Autodesk Fusion 360 part; units mm, degrees
note: some values were not read from the file. Set by a fixed rule: the direction of a hole.
(part 3 of 10)
  line L1913 (9.2464, 17.0934) -> (9.2464, 17.0934)
  line L1914 (9.1415, 16.1798) -> (9.1415, 16.1798)
  line L1915 (9.1415, 16.8402) -> (9.1415, 16.8402)
  line L1916 (10.7434, 17.4236) -> (10.6273, 17.5013)
  line L1917 (11.1785, 16.1798) -> (11.1785, 16.1798)
  line L1918 (9.1415, 16.8402) -> (9.1415, 16.1798)
  line L1919 (9.1415, 16.1798) -> (9.1687, 16.0427)
  line L1920 (9.1687, 16.0427) -> (9.2464, 15.9266)
  line L1921 (9.2464, 15.9266) -> (9.2464, 15.9266)
  line L1922 (46.9384, 15.5964) -> (46.9384, 15.5964)
  line L1923 (46.0248, 17.5285) -> (45.8877, 17.5013)
  line L1924 (45.8877, 17.5013) -> (45.7716, 17.4236)
  line L1925 (47.3463, 16.0427) -> (47.3735, 16.1798)
  line L1926 (46.6852, 17.5285) -> (46.6852, 17.5285)
  line L1927 (46.9384, 17.4236) -> (46.8223, 17.5013)
  line L1928 (47.2686, 17.0934) -> (47.2686, 17.0934)
  line L1929 (47.2686, 15.9266) -> (47.3463, 16.0427)
  line L1930 (45.3365, 16.8402) -> (45.3365, 16.8402)
  line L1931 (46.0248, 15.4915) -> (46.6852, 15.4915)
  line L1932 (47.3735, 16.1798) -> (47.3735, 16.8402)
  line L1933 (45.7716, 17.4236) -> (45.4414, 17.0934)
  line L1934 (45.7716, 15.5964) -> (45.8877, 15.5187)
  line L1935 (45.7716, 17.4236) -> (45.7716, 17.4236)
  line L1936 (46.0248, 15.4915) -> (46.0248, 15.4915)
  line L1937 (45.3365, 16.1798) -> (45.3365, 16.1798)
  line L1938 (46.6852, 15.4915) -> (46.6852, 15.4915)
  line L1939 (46.6852, 17.5285) -> (46.0248, 17.5285)
  line L1940 (46.8223, 17.5013) -> (46.6852, 17.5285)
  line L1941 (45.3637, 16.9773) -> (45.3365, 16.8402)
  line L1942 (46.9384, 15.5964) -> (47.2686, 15.9266)
  line L1943 (47.3463, 16.9773) -> (47.2686, 17.0934)
  line L1944 (47.2686, 17.0934) -> (46.9384, 17.4236)
  line L1945 (46.0248, 17.5285) -> (46.0248, 17.5285)
  line L1946 (45.3365, 16.1798) -> (45.3637, 16.0427)
  line L1947 (45.4414, 17.0934) -> (45.4414, 17.0934)
  line L1948 (45.4414, 17.0934) -> (45.3637, 16.9773)
  line L1949 (47.3735, 16.8402) -> (47.3463, 16.9773)
  line L1950 (45.3637, 16.0427) -> (45.4414, 15.9266)
  line L1951 (46.6852, 15.4915) -> (46.8223, 15.5187)
  line L1952 (45.3365, 16.8402) -> (45.3365, 16.1798)
  line L1953 (47.3735, 16.1798) -> (47.3735, 16.1798)
  line L1954 (45.8877, 15.5187) -> (46.0248, 15.4915)
  line L1955 (46.8223, 15.5187) -> (46.9384, 15.5964)
  line L1956 (47.3735, 16.8402) -> (47.3735, 16.8402)
  line L1957 (46.9384, 17.4236) -> (46.9384, 17.4236)
  line L1958 (47.2686, 15.9266) -> (47.2686, 15.9266)
  line L1959 (45.4414, 15.9266) -> (45.4414, 15.9266)
  line L1960 (45.4414, 15.9266) -> (45.7716, 15.5964)
  line L1961 (45.7716, 15.5964) -> (45.7716, 15.5964)
  line L1962 (11.0736, 29.8966) -> (11.0736, 29.8966)
  line L1963 (10.7434, 29.5664) -> (11.0736, 29.8966)
  line L1964 (11.0736, 31.0634) -> (11.0736, 31.0634)
  line L1965 (10.7434, 29.5664) -> (10.7434, 29.5664)
  line L1966 (11.1785, 30.8102) -> (11.1785, 30.8102)
  line L1967 (9.1415, 30.1498) -> (9.1415, 30.1498)
  line L1968 (10.7434, 31.3936) -> (10.7434, 31.3936)
  line L1969 (9.5766, 31.3936) -> (9.5766, 31.3936)
  line L1970 (9.5766, 31.3936) -> (9.2464, 31.0634)
  line L1971 (10.6273, 31.4713) -> (10.4902, 31.4985)
  line L1972 (10.4902, 31.4985) -> (10.4902, 31.4985)
  line L1973 (9.2464, 31.0634) -> (9.2464, 31.0634)
  line L1974 (9.8298, 31.4985) -> (9.6927, 31.4713)
  line L1975 (9.1415, 30.1498) -> (9.1687, 30.0127)
  line L1976 (9.2464, 29.8966) -> (9.2464, 29.8966)
  line L1977 (11.1513, 30.0127) -> (11.1785, 30.1498)
  line L1978 (9.1687, 30.0127) -> (9.2464, 29.8966)
  line L1979 (9.1415, 30.8102) -> (9.1415, 30.1498)
  line L1980 (11.0736, 29.8966) -> (11.1513, 30.0127)
  line L1981 (11.1785, 30.1498) -> (11.1785, 30.1498)
  line L1982 (10.4902, 31.4985) -> (9.8298, 31.4985)
  line L1983 (9.2464, 31.0634) -> (9.1687, 30.9473)
  line L1984 (10.7434, 31.3936) -> (10.6273, 31.4713)
  line L1985 (9.8298, 31.4985) -> (9.8298, 31.4985)
  line L1986 (9.6927, 31.4713) -> (9.5766, 31.3936)
  line L1987 (9.1415, 30.8102) -> (9.1415, 30.8102)
  line L1988 (9.1687, 30.9473) -> (9.1415, 30.8102)
  line L1989 (11.0736, 31.0634) -> (10.7434, 31.3936)
  line L1990 (9.5766, 29.5664) -> (9.5766, 29.5664)
  line L1991 (9.2464, 29.8966) -> (9.5766, 29.5664)
  line L1992 (10.6273, 29.4887) -> (10.7434, 29.5664)
  line L1993 (9.5766, 29.5664) -> (9.6927, 29.4887)
  line L1994 (10.4902, 29.4615) -> (10.4902, 29.4615)
  line L1995 (9.8298, 29.4615) -> (10.4902, 29.4615)
  line L1996 (9.8298, 29.4615) -> (9.8298, 29.4615)
  line L1997 (9.6927, 29.4887) -> (9.8298, 29.4615)
  line L1998 (10.4902, 29.4615) -> (10.6273, 29.4887)
  line L1999 (11.1513, 30.9473) -> (11.0736, 31.0634)
  line L2000 (11.1785, 30.8102) -> (11.1513, 30.9473)
  line L2001 (11.1785, 30.1498) -> (11.1785, 30.8102)
  line L2002 (56.1315, 16.8402) -> (56.1315, 16.8402)
  line L2003 (56.5666, 17.4236) -> (56.5666, 17.4236)
  line L2004 (56.5666, 17.4236) -> (56.2364, 17.0934)
  line L2005 (56.8198, 17.5285) -> (56.6827, 17.5013)
  line L2006 (57.6173, 15.5187) -> (57.7334, 15.5964)
  line L2007 (58.1685, 16.1798) -> (58.1685, 16.1798)
  line L2008 (58.0636, 17.0934) -> (57.7334, 17.4236)
  line L2009 (57.7334, 17.4236) -> (57.7334, 17.4236)
  line L2010 (56.8198, 17.5285) -> (56.8198, 17.5285)
  line L2011 (57.6173, 17.5013) -> (57.4802, 17.5285)
  line L2012 (58.0636, 15.9266) -> (58.0636, 15.9266)
  line L2013 (56.2364, 17.0934) -> (56.1587, 16.9773)
  line L2014 (56.1315, 16.1798) -> (56.1587, 16.0427)
  line L2015 (56.1315, 16.1798) -> (56.1315, 16.1798)
  line L2016 (57.7334, 17.4236) -> (57.6173, 17.5013)
  line L2017 (57.7334, 15.5964) -> (58.0636, 15.9266)
  line L2018 (58.1685, 16.8402) -> (58.1685, 16.8402)
  line L2019 (58.1685, 16.1798) -> (58.1685, 16.8402)
  line L2020 (56.8198, 15.4915) -> (57.4802, 15.4915)
  line L2021 (58.1685, 16.8402) -> (58.1413, 16.9773)
  line L2022 (58.1413, 16.9773) -> (58.0636, 17.0934)
  line L2023 (58.0636, 15.9266) -> (58.1413, 16.0427)
  line L2024 (58.0636, 17.0934) -> (58.0636, 17.0934)
  line L2025 (58.1413, 16.0427) -> (58.1685, 16.1798)
  line L2026 (57.4802, 15.4915) -> (57.6173, 15.5187)
  line L2027 (57.4802, 15.4915) -> (57.4802, 15.4915)
  line L2028 (56.1315, 16.8402) -> (56.1315, 16.1798)
  line L2029 (56.1587, 16.9773) -> (56.1315, 16.8402)
  line L2030 (56.1587, 16.0427) -> (56.2364, 15.9266)
  line L2031 (56.2364, 17.0934) -> (56.2364, 17.0934)
  line L2032 (57.4802, 17.5285) -> (56.8198, 17.5285)
  line L2033 (56.6827, 15.5187) -> (56.8198, 15.4915)
  line L2034 (56.6827, 17.5013) -> (56.5666, 17.4236)
  line L2035 (56.5666, 15.5964) -> (56.6827, 15.5187)
  line L2036 (56.5666, 15.5964) -> (56.5666, 15.5964)
  line L2037 (57.7334, 15.5964) -> (57.7334, 15.5964)
  line L2038 (56.8198, 15.4915) -> (56.8198, 15.4915)
  line L2039 (56.2364, 15.9266) -> (56.5666, 15.5964)
  line L2040 (57.4802, 17.5285) -> (57.4802, 17.5285)
  line L2041 (56.2364, 15.9266) -> (56.2364, 15.9266)
  line L2042 (21.8687, 19.8527) -> (21.9464, 19.7366)
  line L2043 (21.9464, 20.9034) -> (21.9464, 20.9034)
  line L2044 (22.2766, 21.2336) -> (21.9464, 20.9034)
  line L2045 (21.9464, 20.9034) -> (21.8687, 20.7873)
  line L2046 (22.3927, 21.3113) -> (22.2766, 21.2336)
  line L2047 (22.2766, 21.2336) -> (22.2766, 21.2336)
  line L2048 (23.4434, 21.2336) -> (23.3273, 21.3113)
  line L2049 (22.5298, 21.3385) -> (22.3927, 21.3113)
  line L2050 (23.7736, 20.9034) -> (23.7736, 20.9034)
  line L2051 (22.2766, 19.4064) -> (22.3927, 19.3287)
  line L2052 (22.5298, 19.3015) -> (22.5298, 19.3015)
  line L2053 (23.7736, 20.9034) -> (23.4434, 21.2336)
  line L2054 (23.7736, 19.7366) -> (23.8513, 19.8527)
  line L2055 (23.8785, 19.9898) -> (23.8785, 20.6502)
  line L2056 (23.7736, 19.7366) -> (23.7736, 19.7366)
  line L2057 (22.3927, 19.3287) -> (22.5298, 19.3015)
  line L2058 (23.8785, 20.6502) -> (23.8785, 20.6502)
  line L2059 (21.9464, 19.7366) -> (21.9464, 19.7366)
  line L2060 (21.8415, 20.6502) -> (21.8415, 20.6502)
  line L2061 (21.8415, 19.9898) -> (21.8415, 19.9898)
  line L2062 (21.8687, 20.7873) -> (21.8415, 20.6502)
  line L2063 (23.8513, 19.8527) -> (23.8785, 19.9898)
  line L2064 (23.1902, 19.3015) -> (23.1902, 19.3015)
  line L2065 (22.2766, 19.4064) -> (22.2766, 19.4064)
  line L2066 (21.9464, 19.7366) -> (22.2766, 19.4064)
  line L2067 (22.5298, 19.3015) -> (23.1902, 19.3015)
  line L2068 (23.1902, 21.3385) -> (23.1902, 21.3385)
  line L2069 (23.1902, 21.3385) -> (22.5298, 21.3385)
  line L2070 (23.3273, 21.3113) -> (23.1902, 21.3385)
  line L2071 (23.1902, 19.3015) -> (23.3273, 19.3287)
  line L2072 (21.8415, 20.6502) -> (21.8415, 19.9898)
  line L2073 (21.8415, 19.9898) -> (21.8687, 19.8527)
  line L2074 (22.5298, 21.3385) -> (22.5298, 21.3385)
  line L2075 (23.4434, 19.4064) -> (23.7736, 19.7366)
  line L2076 (23.8513, 20.7873) -> (23.7736, 20.9034)
  line L2077 (23.3273, 19.3287) -> (23.4434, 19.4064)
  line L2078 (23.4434, 19.4064) -> (23.4434, 19.4064)
  line L2079 (23.8785, 19.9898) -> (23.8785, 19.9898)
  line L2080 (23.8785, 20.6502) -> (23.8513, 20.7873)
  line L2081 (23.4434, 21.2336) -> (23.4434, 21.2336)
  line L2082 (36.0273, 17.5013) -> (35.8902, 17.5285)
  line L2083 (35.8902, 17.5285) -> (35.2298, 17.5285)
  line L2084 (34.5415, 16.1798) -> (34.5687, 16.0427)
  line L2085 (34.5415, 16.8402) -> (34.5415, 16.1798)
  line L2086 (34.5415, 16.1798) -> (34.5415, 16.1798)
  line L2087 (34.5687, 16.9773) -> (34.5415, 16.8402)
  line L2088 (35.8902, 15.4915) -> (36.0273, 15.5187)
  line L2089 (35.2298, 15.4915) -> (35.2298, 15.4915)
  line L2090 (35.2298, 15.4915) -> (35.8902, 15.4915)
  line L2091 (35.8902, 15.4915) -> (35.8902, 15.4915)
  line L2092 (36.1434, 15.5964) -> (36.1434, 15.5964)
  line L2093 (36.4736, 17.0934) -> (36.4736, 17.0934)
  line L2094 (34.9766, 15.5964) -> (35.0927, 15.5187)
  line L2095 (36.0273, 15.5187) -> (36.1434, 15.5964)
  line L2096 (36.5513, 16.0427) -> (36.5785, 16.1798)
  line L2097 (36.1434, 15.5964) -> (36.4736, 15.9266)
  line L2098 (36.5785, 16.1798) -> (36.5785, 16.8402)
  line L2099 (36.4736, 15.9266) -> (36.4736, 15.9266)
  line L2100 (36.4736, 15.9266) -> (36.5513, 16.0427)
  line L2101 (36.1434, 17.4236) -> (36.0273, 17.5013)
  line L2102 (35.0927, 15.5187) -> (35.2298, 15.4915)
  line L2103 (34.5687, 16.0427) -> (34.6464, 15.9266)
  line L2104 (34.6464, 17.0934) -> (34.5687, 16.9773)
  line L2105 (34.9766, 15.5964) -> (34.9766, 15.5964)
  line L2106 (35.8902, 17.5285) -> (35.8902, 17.5285)
  line L2107 (36.5785, 16.1798) -> (36.5785, 16.1798)
  line L2108 (36.4736, 17.0934) -> (36.1434, 17.4236)
  line L2109 (35.2298, 17.5285) -> (35.2298, 17.5285)
  line L2110 (35.0927, 17.5013) -> (34.9766, 17.4236)
  line L2111 (36.5785, 16.8402) -> (36.5785, 16.8402)
  line L2112 (34.9766, 17.4236) -> (34.6464, 17.0934)
  line L2113 (36.1434, 17.4236) -> (36.1434, 17.4236)
  line L2114 (34.9766, 17.4236) -> (34.9766, 17.4236)
  line L2115 (36.5513, 16.9773) -> (36.4736, 17.0934)
  line L2116 (36.5785, 16.8402) -> (36.5513, 16.9773)
  line L2117 (34.6464, 17.0934) -> (34.6464, 17.0934)
  line L2118 (34.5415, 16.8402) -> (34.5415, 16.8402)
  line L2119 (34.6464, 15.9266) -> (34.9766, 15.5964)
  line L2120 (34.6464, 15.9266) -> (34.6464, 15.9266)
  line L2121 (35.2298, 17.5285) -> (35.0927, 17.5013)
  line L2122 (11.0736, 19.7366) -> (11.1513, 19.8527)
  line L2123 (10.7434, 21.2336) -> (10.6273, 21.3113)
  line L2124 (10.7434, 21.2336) -> (10.7434, 21.2336)
  line L2125 (9.1415, 19.9898) -> (9.1687, 19.8527)
  line L2126 (9.2464, 20.9034) -> (9.2464, 20.9034)
  line L2127 (10.6273, 21.3113) -> (10.4902, 21.3385)
  line L2128 (11.1785, 19.9898) -> (11.1785, 20.6502)
  line L2129 (11.1785, 20.6502) -> (11.1513, 20.7873)
  line L2130 (10.7434, 19.4064) -> (10.7434, 19.4064)
  line L2131 (9.8298, 21.3385) -> (9.8298, 21.3385)
  line L2132 (9.1687, 19.8527) -> (9.2464, 19.7366)
  line L2133 (11.1513, 20.7873) -> (11.0736, 20.9034)
  line L2134 (9.8298, 19.3015) -> (10.4902, 19.3015)
  line L2135 (9.2464, 19.7366) -> (9.5766, 19.4064)
  line L2136 (10.4902, 19.3015) -> (10.4902, 19.3015)
  line L2137 (10.4902, 19.3015) -> (10.6273, 19.3287)
  line L2138 (9.8298, 21.3385) -> (9.6927, 21.3113)
  line L2139 (9.1415, 20.6502) -> (9.1415, 19.9898)
  line L2140 (10.6273, 19.3287) -> (10.7434, 19.4064)
  line L2141 (9.5766, 21.2336) -> (9.2464, 20.9034)
  line L2142 (11.1785, 20.6502) -> (11.1785, 20.6502)
  line L2143 (9.1415, 20.6502) -> (9.1415, 20.6502)
  line L2144 (10.4902, 21.3385) -> (9.8298, 21.3385)
  line L2145 (10.7434, 19.4064) -> (11.0736, 19.7366)
  line L2146 (11.0736, 19.7366) -> (11.0736, 19.7366)
  line L2147 (11.1513, 19.8527) -> (11.1785, 19.9898)
  line L2148 (11.0736, 20.9034) -> (11.0736, 20.9034)
  line L2149 (9.5766, 19.4064) -> (9.6927, 19.3287)
  line L2150 (10.4902, 21.3385) -> (10.4902, 21.3385)
  line L2151 (9.1687, 20.7873) -> (9.1415, 20.6502)
  line L2152 (9.6927, 19.3287) -> (9.8298, 19.3015)
  line L2153 (9.6927, 21.3113) -> (9.5766, 21.2336)
  line L2154 (9.5766, 21.2336) -> (9.5766, 21.2336)
  line L2155 (9.1415, 19.9898) -> (9.1415, 19.9898)
  line L2156 (11.1785, 19.9898) -> (11.1785, 19.9898)
  line L2157 (9.2464, 20.9034) -> (9.1687, 20.7873)
  line L2158 (9.2464, 19.7366) -> (9.2464, 19.7366)
  line L2159 (11.0736, 20.9034) -> (10.7434, 21.2336)
  line L2160 (9.8298, 19.3015) -> (9.8298, 19.3015)
  line L2161 (9.5766, 19.4064) -> (9.5766, 19.4064)
  line L2162 (21.0066, 77.7486) -> (21.0066, 77.7486)
  line L2163 (21.2598, 77.8535) -> (21.2598, 77.8535)
  line L2164 (21.2598, 75.8165) -> (21.2598, 75.8165)
  line L2165 (21.9202, 75.8165) -> (21.9202, 75.8165)
  line L2166 (22.6085, 76.5048) -> (22.6085, 76.5048)
  line L2167 (22.6085, 76.5048) -> (22.6085, 77.1652)
  line L2168 (22.5813, 77.3023) -> (22.5036, 77.4184)
  line L2169 (22.1734, 77.7486) -> (22.1734, 77.7486)
  line L2170 (21.1227, 75.8437) -> (21.2598, 75.8165)
  line L2171 (21.9202, 75.8165) -> (22.0573, 75.8437)
  line L2172 (22.1734, 77.7486) -> (22.0573, 77.8263)
  line L2173 (20.5987, 77.3023) -> (20.5715, 77.1652)
  line L2174 (21.9202, 77.8535) -> (21.2598, 77.8535)
  line L2175 (21.2598, 75.8165) -> (21.9202, 75.8165)
  line L2176 (20.6764, 77.4184) -> (20.6764, 77.4184)
  line L2177 (22.1734, 75.9214) -> (22.5036, 76.2516)
  line L2178 (22.1734, 75.9214) -> (22.1734, 75.9214)
  line L2179 (21.0066, 75.9214) -> (21.1227, 75.8437)
  line L2180 (22.5036, 77.4184) -> (22.5036, 77.4184)
  line L2181 (21.9202, 77.8535) -> (21.9202, 77.8535)
  line L2182 (20.5715, 76.5048) -> (20.5715, 76.5048)
  line L2183 (20.6764, 76.2516) -> (20.6764, 76.2516)
  line L2184 (22.0573, 75.8437) -> (22.1734, 75.9214)
  line L2185 (22.5036, 76.2516) -> (22.5036, 76.2516)
  line L2186 (20.5987, 76.3677) -> (20.6764, 76.2516)
  line L2187 (22.6085, 77.1652) -> (22.6085, 77.1652)
  line L2188 (22.5036, 76.2516) -> (22.5813, 76.3677)
  line L2189 (22.5036, 77.4184) -> (22.1734, 77.7486)
  line L2190 (21.1227, 77.8263) -> (21.0066, 77.7486)
  line L2191 (21.2598, 77.8535) -> (21.1227, 77.8263)
  line L2192 (20.6764, 76.2516) -> (21.0066, 75.9214)
  line L2193 (21.0066, 75.9214) -> (21.0066, 75.9214)
  line L2194 (22.6085, 77.1652) -> (22.5813, 77.3023)
  line L2195 (21.0066, 77.7486) -> (20.6764, 77.4184)
  line L2196 (22.0573, 77.8263) -> (21.9202, 77.8535)
  line L2197 (20.5715, 77.1652) -> (20.5715, 76.5048)
  line L2198 (20.5715, 76.5048) -> (20.5987, 76.3677)
  line L2199 (20.5715, 77.1652) -> (20.5715, 77.1652)
  line L2200 (22.5813, 76.3677) -> (22.6085, 76.5048)
  line L2201 (20.6764, 77.4184) -> (20.5987, 77.3023)
  line L2202 (23.8513, 30.0127) -> (23.8785, 30.1498)
  line L2203 (21.9464, 29.8966) -> (22.2766, 29.5664)
  line L2204 (22.2766, 31.3936) -> (22.2766, 31.3936)
  line L2205 (21.9464, 31.0634) -> (21.8687, 30.9473)
  line L2206 (22.2766, 29.5664) -> (22.2766, 29.5664)
  line L2207 (21.8415, 30.8102) -> (21.8415, 30.8102)
  line L2208 (21.8687, 30.9473) -> (21.8415, 30.8102)
  line L2209 (21.8415, 30.1498) -> (21.8415, 30.1498)
  line L2210 (22.2766, 31.3936) -> (21.9464, 31.0634)
  line L2211 (22.5298, 31.4985) -> (22.3927, 31.4713)
  line L2212 (22.3927, 31.4713) -> (22.2766, 31.3936)
  line L2213 (23.8513, 30.9473) -> (23.7736, 31.0634)
  line L2214 (21.8415, 30.8102) -> (21.8415, 30.1498)
  line L2215 (21.9464, 29.8966) -> (21.9464, 29.8966)
  line L2216 (21.8415, 30.1498) -> (21.8687, 30.0127)
  line L2217 (21.8687, 30.0127) -> (21.9464, 29.8966)
  line L2218 (21.9464, 31.0634) -> (21.9464, 31.0634)
  line L2219 (22.5298, 31.4985) -> (22.5298, 31.4985)
  line L2220 (22.5298, 29.4615) -> (23.1902, 29.4615)
  line L2221 (23.8785, 30.1498) -> (23.8785, 30.8102)
  line L2222 (23.1902, 29.4615) -> (23.3273, 29.4887)
  line L2223 (23.7736, 31.0634) -> (23.7736, 31.0634)
  line L2224 (23.4434, 31.3936) -> (23.4434, 31.3936)
  line L2225 (23.4434, 31.3936) -> (23.3273, 31.4713)
  line L2226 (23.1902, 29.4615) -> (23.1902, 29.4615)
  line L2227 (23.1902, 31.4985) -> (22.5298, 31.4985)
  line L2228 (23.4434, 29.5664) -> (23.4434, 29.5664)
  line L2229 (23.3273, 31.4713) -> (23.1902, 31.4985)
  line L2230 (23.7736, 29.8966) -> (23.7736, 29.8966)
  line L2231 (23.8785, 30.8102) -> (23.8785, 30.8102)
  line L2232 (23.8785, 30.8102) -> (23.8513, 30.9473)
  line L2233 (23.4434, 29.5664) -> (23.7736, 29.8966)
  line L2234 (23.3273, 29.4887) -> (23.4434, 29.5664)
  line L2235 (23.7736, 31.0634) -> (23.4434, 31.3936)
  line L2236 (23.1902, 31.4985) -> (23.1902, 31.4985)
  line L2237 (22.5298, 29.4615) -> (22.5298, 29.4615)
  line L2238 (23.8785, 30.1498) -> (23.8785, 30.1498)
  line L2239 (22.2766, 29.5664) -> (22.3927, 29.4887)
  line L2240 (23.7736, 29.8966) -> (23.8513, 30.0127)
  line L2241 (22.3927, 29.4887) -> (22.5298, 29.4615)
  line L2242 (28.6266, 75.9214) -> (28.7427, 75.8437)
  line L2243 (28.7427, 75.8437) -> (28.8798, 75.8165)
  line L2244 (30.2285, 76.5048) -> (30.2285, 76.5048)
  line L2245 (29.5402, 77.8535) -> (28.8798, 77.8535)
  line L2246 (30.1236, 76.2516) -> (30.2013, 76.3677)
  line L2247 (28.1915, 76.5048) -> (28.2187, 76.3677)
  line L2248 (28.8798, 77.8535) -> (28.8798, 77.8535)
  line L2249 (28.1915, 76.5048) -> (28.1915, 76.5048)
  line L2250 (28.8798, 75.8165) -> (29.5402, 75.8165)
  line L2251 (28.1915, 77.1652) -> (28.1915, 76.5048)
  line L2252 (29.7934, 75.9214) -> (30.1236, 76.2516)
  line L2253 (30.2285, 76.5048) -> (30.2285, 77.1652)
  line L2254 (29.7934, 75.9214) -> (29.7934, 75.9214)
  line L2255 (29.5402, 75.8165) -> (29.5402, 75.8165)
  line L2256 (29.7934, 77.7486) -> (29.6773, 77.8263)
  line L2257 (30.2285, 77.1652) -> (30.2013, 77.3023)
  line L2258 (29.5402, 77.8535) -> (29.5402, 77.8535)
  line L2259 (30.2013, 76.3677) -> (30.2285, 76.5048)
  line L2260 (28.6266, 77.7486) -> (28.2964, 77.4184)
  line L2261 (29.7934, 77.7486) -> (29.7934, 77.7486)
  line L2262 (28.2187, 77.3023) -> (28.1915, 77.1652)
  line L2263 (29.5402, 75.8165) -> (29.6773, 75.8437)
  line L2264 (28.2187, 76.3677) -> (28.2964, 76.2516)
  line L2265 (28.2964, 77.4184) -> (28.2964, 77.4184)
  line L2266 (28.8798, 77.8535) -> (28.7427, 77.8263)
  line L2267 (28.7427, 77.8263) -> (28.6266, 77.7486)
  line L2268 (29.6773, 75.8437) -> (29.7934, 75.9214)
  line L2269 (30.1236, 76.2516) -> (30.1236, 76.2516)
  line L2270 (30.1236, 77.4184) -> (30.1236, 77.4184)
  line L2271 (28.8798, 75.8165) -> (28.8798, 75.8165)
  line L2272 (30.2285, 77.1652) -> (30.2285, 77.1652)
  line L2273 (28.2964, 76.2516) -> (28.2964, 76.2516)
  line L2274 (28.1915, 77.1652) -> (28.1915, 77.1652)
  line L2275 (30.1236, 77.4184) -> (29.7934, 77.7486)
  line L2276 (29.6773, 77.8263) -> (29.5402, 77.8535)
  line L2277 (28.2964, 76.2516) -> (28.6266, 75.9214)
  line L2278 (28.6266, 77.7486) -> (28.6266, 77.7486)
  line L2279 (28.2964, 77.4184) -> (28.2187, 77.3023)
  line L2280 (30.2013, 77.3023) -> (30.1236, 77.4184)
  line L2281 (21.9464, 15.9266) -> (21.9464, 15.9266)
  line L2282 (21.8415, 16.8402) -> (21.8415, 16.1798)
  line L2283 (23.3273, 17.5013) -> (23.1902, 17.5285)
  line L2284 (23.1902, 17.5285) -> (22.5298, 17.5285)
  line L2285 (21.8415, 16.8402) -> (21.8415, 16.8402)
  line L2286 (21.9464, 15.9266) -> (22.2766, 15.5964)
  line L2287 (23.4434, 15.5964) -> (23.4434, 15.5964)
  line L2288 (23.4434, 15.5964) -> (23.7736, 15.9266)
  line L2289 (22.2766, 15.5964) -> (22.3927, 15.5187)
  line L2290 (23.4434, 17.4236) -> (23.4434, 17.4236)
  line L2291 (23.8785, 16.8402) -> (23.8785, 16.8402)
  line L2292 (23.7736, 15.9266) -> (23.7736, 15.9266)
  line L2293 (23.8785, 16.1798) -> (23.8785, 16.1798)
  line L2294 (23.8513, 16.0427) -> (23.8785, 16.1798)
  line L2295 (23.4434, 17.4236) -> (23.3273, 17.5013)
  line L2296 (22.5298, 17.5285) -> (22.3927, 17.5013)
  line L2297 (23.7736, 15.9266) -> (23.8513, 16.0427)
  line L2298 (21.9464, 17.0934) -> (21.9464, 17.0934)
  line L2299 (23.8785, 16.1798) -> (23.8785, 16.8402)
  line L2300 (23.1902, 17.5285) -> (23.1902, 17.5285)
  line L2301 (22.5298, 17.5285) -> (22.5298, 17.5285)
  line L2302 (22.3927, 17.5013) -> (22.2766, 17.4236)
  line L2303 (22.5298, 15.4915) -> (22.5298, 15.4915)
  line L2304 (22.3927, 15.5187) -> (22.5298, 15.4915)
  line L2305 (23.1902, 15.4915) -> (23.3273, 15.5187)
  line L2306 (23.3273, 15.5187) -> (23.4434, 15.5964)
  line L2307 (22.5298, 15.4915) -> (23.1902, 15.4915)
  line L2308 (23.1902, 15.4915) -> (23.1902, 15.4915)
  line L2309 (23.8785, 16.8402) -> (23.8513, 16.9773)
  line L2310 (23.8513, 16.9773) -> (23.7736, 17.0934)
  line L2311 (23.7736, 17.0934) -> (23.7736, 17.0934)
  line L2312 (23.7736, 17.0934) -> (23.4434, 17.4236)
  line L2313 (22.2766, 15.5964) -> (22.2766, 15.5964)
  line L2314 (21.9464, 17.0934) -> (21.8687, 16.9773)
  line L2315 (21.8687, 16.9773) -> (21.8415, 16.8402)
  line L2316 (22.2766, 17.4236) -> (22.2766, 17.4236)
  line L2317 (21.8415, 16.1798) -> (21.8687, 16.0427)
  line L2318 (21.8415, 16.1798) -> (21.8415, 16.1798)
  line L2319 (21.8687, 16.0427) -> (21.9464, 15.9266)
  line L2320 (22.2766, 17.4236) -> (21.9464, 17.0934)
  line L2321 (88.1416, 17.3518) -> (88.0584, 17.4074)
  line L2322 (87.2998, 17.4269) -> (87.2998, 17.4269)
  line L2323 (87.9602, 15.5931) -> (88.0584, 15.6126)
  line L2324 (88.4718, 17.0216) -> (88.1416, 17.3518)
  line L2325 (87.9602, 17.4269) -> (87.2998, 17.4269)
  line L2326 (88.0584, 15.6126) -> (88.1416, 15.6682)
  line L2327 (88.5469, 16.8402) -> (88.5274, 16.9384)
  line L2328 (88.4718, 17.0216) -> (88.4718, 17.0216)
  line L2329 (87.2998, 15.5931) -> (87.2998, 15.5931)
  line L2330 (86.7882, 15.9984) -> (86.7882, 15.9984)
  line L2331 (86.7882, 17.0216) -> (86.7882, 17.0216)
  line L2332 (86.7326, 16.0816) -> (86.7882, 15.9984)
  line L2333 (88.1416, 15.6682) -> (88.4718, 15.9984)
  line L2334 (88.5469, 16.1798) -> (88.5469, 16.8402)
  line L2335 (87.2016, 15.6126) -> (87.2998, 15.5931)
  line L2336 (86.7882, 17.0216) -> (86.7326, 16.9384)
  line L2337 (86.7131, 16.1798) -> (86.7326, 16.0816)
  line L2338 (86.7131, 16.8402) -> (86.7131, 16.1798)
  line L2339 (88.5274, 16.9384) -> (88.4718, 17.0216)
  line L2340 (86.7131, 16.8402) -> (86.7131, 16.8402)
  line L2341 (88.5469, 16.1798) -> (88.5469, 16.1798)
  line L2342 (86.7326, 16.9384) -> (86.7131, 16.8402)
  line L2343 (87.1184, 17.3518) -> (87.1184, 17.3518)
  line L2344 (87.2016, 17.4074) -> (87.1184, 17.3518)
  line L2345 (87.2998, 17.4269) -> (87.2016, 17.4074)
  line L2346 (87.1184, 17.3518) -> (86.7882, 17.0216)
  line L2347 (88.4718, 15.9984) -> (88.4718, 15.9984)
  line L2348 (88.0584, 17.4074) -> (87.9602, 17.4269)
  line L2349 (88.1416, 17.3518) -> (88.1416, 17.3518)
  line L2350 (87.9602, 17.4269) -> (87.9602, 17.4269)
  line L2351 (88.5274, 16.0816) -> (88.5469, 16.1798)
  line L2352 (88.4718, 15.9984) -> (88.5274, 16.0816)
  line L2353 (87.1184, 15.6682) -> (87.1184, 15.6682)
  line L2354 (86.7882, 15.9984) -> (87.1184, 15.6682)
  line L2355 (87.1184, 15.6682) -> (87.2016, 15.6126)
  line L2356 (88.1416, 15.6682) -> (88.1416, 15.6682)
  line L2357 (87.2998, 15.5931) -> (87.9602, 15.5931)
  line L2358 (86.7131, 16.1798) -> (86.7131, 16.1798)
  line L2359 (87.9602, 15.5931) -> (87.9602, 15.5931)
  line L2360 (88.5469, 16.8402) -> (88.5469, 16.8402)
  line L2361 (65.2816, 17.3518) -> (65.2816, 17.3518)
  line L2362 (65.6118, 15.9984) -> (65.6118, 15.9984)
  line L2363 (65.6869, 16.1798) -> (65.6869, 16.8402)
  line L2364 (65.6869, 16.8402) -> (65.6674, 16.9384)
  line L2365 (65.6869, 16.1798) -> (65.6869, 16.1798)
  line L2366 (65.6118, 17.0216) -> (65.6118, 17.0216)
  line L2367 (65.2816, 17.3518) -> (65.1984, 17.4074)
  line L2368 (65.6674, 16.9384) -> (65.6118, 17.0216)
  line L2369 (64.2584, 15.6682) -> (64.3416, 15.6126)
  line L2370 (64.3416, 15.6126) -> (64.4398, 15.5931)
  line L2371 (64.4398, 15.5931) -> (64.4398, 15.5931)
  line L2372 (65.1002, 15.5931) -> (65.1002, 15.5931)
  line L2373 (64.4398, 15.5931) -> (65.1002, 15.5931)
  line L2374 (65.2816, 15.6682) -> (65.2816, 15.6682)
  line L2375 (65.1002, 15.5931) -> (65.1984, 15.6126)
  line L2376 (65.6674, 16.0816) -> (65.6869, 16.1798)
  line L2377 (65.1984, 15.6126) -> (65.2816, 15.6682)
  line L2378 (65.2816, 15.6682) -> (65.6118, 15.9984)
  line L2379 (65.6118, 15.9984) -> (65.6674, 16.0816)
  line L2380 (63.8531, 16.8402) -> (63.8531, 16.1798)
  line L2381 (64.4398, 17.4269) -> (64.3416, 17.4074)
  line L2382 (63.8531, 16.8402) -> (63.8531, 16.8402)
  line L2383 (63.9282, 15.9984) -> (63.9282, 15.9984)
  line L2384 (63.8726, 16.9384) -> (63.8531, 16.8402)
  line L2385 (64.2584, 15.6682) -> (64.2584, 15.6682)
  line L2386 (63.8726, 16.0816) -> (63.9282, 15.9984)
  line L2387 (63.8531, 16.1798) -> (63.8531, 16.1798)
  line L2388 (65.1984, 17.4074) -> (65.1002, 17.4269)
  line L2389 (63.9282, 15.9984) -> (64.2584, 15.6682)
  line L2390 (63.9282, 17.0216) -> (63.8726, 16.9384)
  line L2391 (64.2584, 17.3518) -> (64.2584, 17.3518)
  line L2392 (65.1002, 17.4269) -> (65.1002, 17.4269)
  line L2393 (64.4398, 17.4269) -> (64.4398, 17.4269)
  line L2394 (65.1002, 17.4269) -> (64.4398, 17.4269)
  line L2395 (63.9282, 17.0216) -> (63.9282, 17.0216)
  line L2396 (63.8531, 16.1798) -> (63.8726, 16.0816)
  line L2397 (64.2584, 17.3518) -> (63.9282, 17.0216)
  line L2398 (64.3416, 17.4074) -> (64.2584, 17.3518)
  line L2399 (65.6118, 17.0216) -> (65.2816, 17.3518)
  line L2400 (65.6869, 16.8402) -> (65.6869, 16.8402)
  line L2401 (25.7302, 17.4269) -> (25.7302, 17.4269)
  line L2402 (24.5582, 17.0216) -> (24.5582, 17.0216)
  line L2403 (24.8884, 15.6682) -> (24.8884, 15.6682)
  line L2404 (24.5026, 16.0816) -> (24.5582, 15.9984)
  line L2405 (26.2418, 17.0216) -> (26.2418, 17.0216)
  line L2406 (24.4831, 16.8402) -> (24.4831, 16.8402)
  line L2407 (25.0698, 17.4269) -> (25.0698, 17.4269)
  line L2408 (26.3169, 16.1798) -> (26.3169, 16.1798)
  line L2409 (24.4831, 16.1798) -> (24.4831, 16.1798)
  line L2410 (26.2418, 15.9984) -> (26.2418, 15.9984)
  line L2411 (25.9116, 15.6682) -> (25.9116, 15.6682)
  line L2412 (26.2418, 17.0216) -> (25.9116, 17.3518)
  line L2413 (25.0698, 15.5931) -> (25.0698, 15.5931)
  line L2414 (24.8884, 17.3518) -> (24.5582, 17.0216)
  line L2415 (25.0698, 17.4269) -> (24.9716, 17.4074)
  line L2416 (24.4831, 16.1798) -> (24.5026, 16.0816)
  line L2417 (26.2974, 16.9384) -> (26.2418, 17.0216)
  line L2418 (24.5582, 15.9984) -> (24.8884, 15.6682)
  line L2419 (25.7302, 17.4269) -> (25.0698, 17.4269)
  line L2420 (26.3169, 16.1798) -> (26.3169, 16.8402)
  line L2421 (25.7302, 15.5931) -> (25.8284, 15.6126)
  line L2422 (25.7302, 15.5931) -> (25.7302, 15.5931)
  line L2423 (25.9116, 17.3518) -> (25.9116, 17.3518)
  line L2424 (25.0698, 15.5931) -> (25.7302, 15.5931)
  line L2425 (24.8884, 15.6682) -> (24.9716, 15.6126)
  line L2426 (24.8884, 17.3518) -> (24.8884, 17.3518)
  line L2427 (24.5026, 16.9384) -> (24.4831, 16.8402)
  line L2428 (25.8284, 17.4074) -> (25.7302, 17.4269)
  line L2429 (24.9716, 17.4074) -> (24.8884, 17.3518)
  line L2430 (24.5582, 17.0216) -> (24.5026, 16.9384)
  line L2431 (25.9116, 17.3518) -> (25.8284, 17.4074)
  line L2432 (24.5582, 15.9984) -> (24.5582, 15.9984)
  line L2433 (24.9716, 15.6126) -> (25.0698, 15.5931)
  line L2434 (24.4831, 16.8402) -> (24.4831, 16.1798)
  line L2435 (25.8284, 15.6126) -> (25.9116, 15.6682)
  line L2436 (26.3169, 16.8402) -> (26.3169, 16.8402)
  line L2437 (25.9116, 15.6682) -> (26.2418, 15.9984)
  line L2438 (26.2418, 15.9984) -> (26.2974, 16.0816)
  line L2439 (26.2974, 16.0816) -> (26.3169, 16.1798)
  line L2440 (26.3169, 16.8402) -> (26.2974, 16.9384)
  line L2441 (55.4518, 15.9984) -> (55.4518, 15.9984)
  line L2442 (54.2798, 17.4269) -> (54.1816, 17.4074)
  line L2443 (53.7682, 15.9984) -> (54.0984, 15.6682)
  line L2444 (54.1816, 17.4074) -> (54.0984, 17.3518)
  line L2445 (54.9402, 17.4269) -> (54.2798, 17.4269)
  line L2446 (54.9402, 17.4269) -> (54.9402, 17.4269)
  line L2447 (53.7126, 16.0816) -> (53.7682, 15.9984)
  line L2448 (53.6931, 16.1798) -> (53.7126, 16.0816)
  line L2449 (55.5269, 16.8402) -> (55.5269, 16.8402)
  line L2450 (55.1216, 15.6682) -> (55.4518, 15.9984)
  line L2451 (53.6931, 16.8402) -> (53.6931, 16.8402)
  line L2452 (53.7682, 17.0216) -> (53.7682, 17.0216)
  line L2453 (55.4518, 15.9984) -> (55.5074, 16.0816)
  line L2454 (55.1216, 15.6682) -> (55.1216, 15.6682)
  line L2455 (54.9402, 15.5931) -> (55.0384, 15.6126)
  line L2456 (55.5269, 16.8402) -> (55.5074, 16.9384)
  line L2457 (54.0984, 17.3518) -> (54.0984, 17.3518)
  line L2458 (54.0984, 15.6682) -> (54.1816, 15.6126)
  line L2459 (54.2798, 15.5931) -> (54.9402, 15.5931)
  line L2460 (53.6931, 16.8402) -> (53.6931, 16.1798)
  line L2461 (55.1216, 17.3518) -> (55.1216, 17.3518)
  line L2462 (54.9402, 15.5931) -> (54.9402, 15.5931)
  line L2463 (55.0384, 17.4074) -> (54.9402, 17.4269)
  line L2464 (55.5074, 16.9384) -> (55.4518, 17.0216)
  line L2465 (55.5269, 16.1798) -> (55.5269, 16.8402)
  line L2466 (55.1216, 17.3518) -> (55.0384, 17.4074)
  line L2467 (54.2798, 17.4269) -> (54.2798, 17.4269)
  line L2468 (55.0384, 15.6126) -> (55.1216, 15.6682)
  line L2469 (55.5074, 16.0816) -> (55.5269, 16.1798)
  line L2470 (55.4518, 17.0216) -> (55.4518, 17.0216)
  line L2471 (55.5269, 16.1798) -> (55.5269, 16.1798)
  line L2472 (53.7682, 15.9984) -> (53.7682, 15.9984)
  line L2473 (54.0984, 17.3518) -> (53.7682, 17.0216)
  line L2474 (54.2798, 15.5931) -> (54.2798, 15.5931)
  line L2475 (54.1816, 15.6126) -> (54.2798, 15.5931)
  line L2476 (54.0984, 15.6682) -> (54.0984, 15.6682)
  line L2477 (53.7682, 17.0216) -> (53.7126, 16.9384)
  line L2478 (53.6931, 16.1798) -> (53.6931, 16.1798)
  line L2479 (55.4518, 17.0216) -> (55.1216, 17.3518)
  line L2480 (53.7126, 16.9384) -> (53.6931, 16.8402)
  line L2481 (75.8698, 17.4269) -> (75.7716, 17.4074)
  line L2482 (76.5302, 17.4269) -> (76.5302, 17.4269)
  line L2483 (76.5302, 15.5931) -> (76.5302, 15.5931)
  line L2484 (75.2831, 16.1798) -> (75.3026, 16.0816)
  line L2485 (75.2831, 16.8402) -> (75.2831, 16.8402)
  line L2486 (75.2831, 16.8402) -> (75.2831, 16.1798)
  line L2487 (77.0418, 17.0216) -> (76.7116, 17.3518)
  line L2488 (75.8698, 15.5931) -> (75.8698, 15.5931)
  line L2489 (75.2831, 16.1798) -> (75.2831, 16.1798)
  line L2490 (75.6884, 15.6682) -> (75.7716, 15.6126)
  line L2491 (75.3582, 17.0216) -> (75.3026, 16.9384)
  line L2492 (75.3582, 17.0216) -> (75.3582, 17.0216)
  line L2493 (75.8698, 15.5931) -> (76.5302, 15.5931)
  line L2494 (75.6884, 17.3518) -> (75.3582, 17.0216)
  line L2495 (75.6884, 17.3518) -> (75.6884, 17.3518)
  line L2496 (76.7116, 17.3518) -> (76.6284, 17.4074)
  line L2497 (76.7116, 17.3518) -> (76.7116, 17.3518)
  line L2498 (77.0974, 16.0816) -> (77.1169, 16.1798)
  line L2499 (77.1169, 16.8402) -> (77.0974, 16.9384)
  line L2500 (77.1169, 16.1798) -> (77.1169, 16.1798)
  line L2501 (76.5302, 15.5931) -> (76.6284, 15.6126)
  line L2502 (76.6284, 15.6126) -> (76.7116, 15.6682)
  line L2503 (77.0418, 15.9984) -> (77.0974, 16.0816)
  line L2504 (77.0974, 16.9384) -> (77.0418, 17.0216)
  line L2505 (76.7116, 15.6682) -> (76.7116, 15.6682)
  line L2506 (76.7116, 15.6682) -> (77.0418, 15.9984)
  line L2507 (77.0418, 15.9984) -> (77.0418, 15.9984)
  line L2508 (77.1169, 16.8402) -> (77.1169, 16.8402)
  line L2509 (75.3582, 15.9984) -> (75.6884, 15.6682)
  line L2510 (77.1169, 16.1798) -> (77.1169, 16.8402)
  line L2511 (76.6284, 17.4074) -> (76.5302, 17.4269)
  line L2512 (75.6884, 15.6682) -> (75.6884, 15.6682)
  line L2513 (75.3026, 16.0816) -> (75.3582, 15.9984)
  line L2514 (75.8698, 17.4269) -> (75.8698, 17.4269)
  line L2515 (75.3026, 16.9384) -> (75.2831, 16.8402)
  line L2516 (75.3582, 15.9984) -> (75.3582, 15.9984)
  line L2517 (75.7716, 17.4074) -> (75.6884, 17.3518)
  line L2518 (77.0418, 17.0216) -> (77.0418, 17.0216)
  line L2519 (76.5302, 17.4269) -> (75.8698, 17.4269)
  line L2520 (75.7716, 15.6126) -> (75.8698, 15.5931)
  line L2521 (11.8026, 16.9384) -> (11.7831, 16.8402)
  line L2522 (13.0302, 15.5931) -> (13.0302, 15.5931)
  line L2523 (11.7831, 16.1798) -> (11.8026, 16.0816)
  line L2524 (12.1884, 17.3518) -> (12.1884, 17.3518)
  line L2525 (11.8026, 16.0816) -> (11.8582, 15.9984)
  line L2526 (11.7831, 16.8402) -> (11.7831, 16.1798)
  line L2527 (12.3698, 17.4269) -> (12.3698, 17.4269)
  line L2528 (12.2716, 15.6126) -> (12.3698, 15.5931)
  line L2529 (11.8582, 17.0216) -> (11.8026, 16.9384)
  line L2530 (11.8582, 17.0216) -> (11.8582, 17.0216)
  line L2531 (12.1884, 15.6682) -> (12.1884, 15.6682)
  line L2532 (11.8582, 15.9984) -> (12.1884, 15.6682)
  line L2533 (12.3698, 15.5931) -> (13.0302, 15.5931)
  line L2534 (13.5418, 15.9984) -> (13.5974, 16.0816)
  line L2535 (13.0302, 15.5931) -> (13.1284, 15.6126)
  line L2536 (12.1884, 17.3518) -> (11.8582, 17.0216)
  line L2537 (13.0302, 17.4269) -> (12.3698, 17.4269)
  line L2538 (12.1884, 15.6682) -> (12.2716, 15.6126)
  line L2539 (12.3698, 15.5931) -> (12.3698, 15.5931)
  line L2540 (13.5418, 17.0216) -> (13.5418, 17.0216)
  line L2541 (12.3698, 17.4269) -> (12.2716, 17.4074)
  line L2542 (13.1284, 17.4074) -> (13.0302, 17.4269)
  line L2543 (13.5418, 17.0216) -> (13.2116, 17.3518)
  line L2544 (13.2116, 17.3518) -> (13.1284, 17.4074)
  line L2545 (13.6169, 16.1798) -> (13.6169, 16.8402)
  line L2546 (13.6169, 16.8402) -> (13.5974, 16.9384)
  line L2547 (12.2716, 17.4074) -> (12.1884, 17.3518)
  line L2548 (13.0302, 17.4269) -> (13.0302, 17.4269)
  line L2549 (13.5974, 16.9384) -> (13.5418, 17.0216)
  line L2550 (13.6169, 16.1798) -> (13.6169, 16.1798)
  line L2551 (13.6169, 16.8402) -> (13.6169, 16.8402)
  line L2552 (13.1284, 15.6126) -> (13.2116, 15.6682)
  line L2553 (13.5974, 16.0816) -> (13.6169, 16.1798)
  line L2554 (13.5418, 15.9984) -> (13.5418, 15.9984)
  line L2555 (13.2116, 15.6682) -> (13.2116, 15.6682)
  line L2556 (13.2116, 15.6682) -> (13.5418, 15.9984)
  line L2557 (11.7831, 16.8402) -> (11.7831, 16.8402)
  line L2558 (13.2116, 17.3518) -> (13.2116, 17.3518)
  line L2559 (11.7831, 16.1798) -> (11.7831, 16.1798)
  line L2560 (11.8582, 15.9984) -> (11.8582, 15.9984)
  line L2561 (48.5648, 15.5931) -> (49.2252, 15.5931)
  line L2562 (49.7924, 16.0816) -> (49.8119, 16.1798)
  line L2563 (48.4666, 17.4074) -> (48.3834, 17.3518)
  line L2564 (49.3234, 15.6126) -> (49.4066, 15.6682)
  line L2565 (48.3834, 17.3518) -> (48.3834, 17.3518)
  line L2566 (48.0532, 17.0216) -> (47.9976, 16.9384)
  line L2567 (49.7368, 15.9984) -> (49.7924, 16.0816)
  line L2568 (47.9781, 16.8402) -> (47.9781, 16.1798)
  line L2569 (49.2252, 17.4269) -> (49.2252, 17.4269)
  line L2570 (48.0532, 17.0216) -> (48.0532, 17.0216)
  line L2571 (49.7924, 16.9384) -> (49.7368, 17.0216)
  line L2572 (49.2252, 17.4269) -> (48.5648, 17.4269)
  line L2573 (49.7368, 15.9984) -> (49.7368, 15.9984)
  line L2574 (47.9781, 16.8402) -> (47.9781, 16.8402)
  line L2575 (49.8119, 16.8402) -> (49.7924, 16.9384)
  line L2576 (47.9976, 16.0816) -> (48.0532, 15.9984)
  line L2577 (48.0532, 15.9984) -> (48.0532, 15.9984)
  line L2578 (47.9976, 16.9384) -> (47.9781, 16.8402)
  line L2579 (49.2252, 15.5931) -> (49.3234, 15.6126)
  line L2580 (48.3834, 15.6682) -> (48.4666, 15.6126)
  line L2581 (49.7368, 17.0216) -> (49.7368, 17.0216)
  line L2582 (48.4666, 15.6126) -> (48.5648, 15.5931)
  line L2583 (48.0532, 15.9984) -> (48.3834, 15.6682)
  line L2584 (49.7368, 17.0216) -> (49.4066, 17.3518)
  line L2585 (48.3834, 17.3518) -> (48.0532, 17.0216)
  line L2586 (48.5648, 15.5931) -> (48.5648, 15.5931)
  line L2587 (49.8119, 16.8402) -> (49.8119, 16.8402)
  line L2588 (49.4066, 17.3518) -> (49.4066, 17.3518)
  line L2589 (48.5648, 17.4269) -> (48.4666, 17.4074)
  line L2590 (49.8119, 16.1798) -> (49.8119, 16.1798)
  line L2591 (47.9781, 16.1798) -> (47.9976, 16.0816)
  line L2592 (49.4066, 15.6682) -> (49.7368, 15.9984)
  line L2593 (49.4066, 17.3518) -> (49.3234, 17.4074)
  line L2594 (47.9781, 16.1798) -> (47.9781, 16.1798)
  line L2595 (48.3834, 15.6682) -> (48.3834, 15.6682)
  line L2596 (49.4066, 15.6682) -> (49.4066, 15.6682)
  line L2597 (49.3234, 17.4074) -> (49.2252, 17.4269)
  line L2598 (49.8119, 16.1798) -> (49.8119, 16.8402)
  line L2599 (48.5648, 17.4269) -> (48.5648, 17.4269)
  line L2600 (49.2252, 15.5931) -> (49.2252, 15.5931)
  line L2601 (37.5884, 15.6682) -> (37.6716, 15.6126)
  line L2602 (37.7698, 15.5931) -> (37.7698, 15.5931)
  line L2603 (37.6716, 15.6126) -> (37.7698, 15.5931)
  line L2604 (37.7698, 15.5931) -> (38.4302, 15.5931)
  line L2605 (38.4302, 15.5931) -> (38.4302, 15.5931)
  line L2606 (38.4302, 15.5931) -> (38.5284, 15.6126)
  line L2607 (38.6116, 15.6682) -> (38.9418, 15.9984)
  line L2608 (37.2582, 17.0216) -> (37.2582, 17.0216)
  line L2609 (37.1831, 16.8402) -> (37.1831, 16.8402)
  line L2610 (37.2582, 17.0216) -> (37.2026, 16.9384)
  line L2611 (37.5884, 17.3518) -> (37.5884, 17.3518)
  line L2612 (38.5284, 17.4074) -> (38.4302, 17.4269)
  line L2613 (38.9974, 16.9384) -> (38.9418, 17.0216)
  line L2614 (39.0169, 16.8402) -> (38.9974, 16.9384)
  line L2615 (39.0169, 16.1798) -> (39.0169, 16.1798)
  line L2616 (39.0169, 16.1798) -> (39.0169, 16.8402)
  line L2617 (38.9974, 16.0816) -> (39.0169, 16.1798)
  line L2618 (38.6116, 15.6682) -> (38.6116, 15.6682)
  line L2619 (38.9418, 15.9984) -> (38.9974, 16.0816)
  line L2620 (38.5284, 15.6126) -> (38.6116, 15.6682)
  line L2621 (39.0169, 16.8402) -> (39.0169, 16.8402)
  line L2622 (38.9418, 17.0216) -> (38.9418, 17.0216)
  line L2623 (38.9418, 17.0216) -> (38.6116, 17.3518)
  line L2624 (38.6116, 17.3518) -> (38.5284, 17.4074)
  line L2625 (38.6116, 17.3518) -> (38.6116, 17.3518)
  line L2626 (37.7698, 17.4269) -> (37.6716, 17.4074)
  line L2627 (37.2582, 15.9984) -> (37.5884, 15.6682)
  line L2628 (37.2026, 16.0816) -> (37.2582, 15.9984)
  line L2629 (37.5884, 17.3518) -> (37.2582, 17.0216)
  line L2630 (38.9418, 15.9984) -> (38.9418, 15.9984)
  line L2631 (37.5884, 15.6682) -> (37.5884, 15.6682)
  line L2632 (37.1831, 16.8402) -> (37.1831, 16.1798)
  line L2633 (37.6716, 17.4074) -> (37.5884, 17.3518)
  line L2634 (37.2582, 15.9984) -> (37.2582, 15.9984)
  line L2635 (37.1831, 16.1798) -> (37.1831, 16.1798)
  line L2636 (38.4302, 17.4269) -> (37.7698, 17.4269)
  line L2637 (37.2026, 16.9384) -> (37.1831, 16.8402)
  line L2638 (37.7698, 17.4269) -> (37.7698, 17.4269)
  line L2639 (38.4302, 17.4269) -> (38.4302, 17.4269)
  line L2640 (37.1831, 16.1798) -> (37.2026, 16.0816)
  line L2641 (24.6416, 75.9932) -> (24.6416, 75.9932)
  line L2642 (24.9718, 76.3234) -> (24.9718, 76.3234)
  line L2643 (24.6416, 75.9932) -> (24.9718, 76.3234)
  line L2644 (25.0469, 77.1652) -> (25.0274, 77.2634)
  line L2645 (24.6416, 77.6768) -> (24.6416, 77.6768)
  line L2646 (24.5584, 75.9376) -> (24.6416, 75.9932)
  line L2647 (24.4602, 77.7519) -> (23.7998, 77.7519)
  line L2648 (23.7998, 77.7519) -> (23.7016, 77.7324)
  line L2649 (23.2131, 76.5048) -> (23.2326, 76.4066)
  line L2650 (23.7016, 75.9376) -> (23.7998, 75.9181)
  line L2651 (24.9718, 76.3234) -> (25.0274, 76.4066)
  line L2652 (25.0274, 77.2634) -> (24.9718, 77.3466)
  line L2653 (24.9718, 77.3466) -> (24.9718, 77.3466)
  line L2654 (23.2131, 76.5048) -> (23.2131, 76.5048)
  line L2655 (23.7998, 77.7519) -> (23.7998, 77.7519)
  line L2656 (23.2131, 77.1652) -> (23.2131, 76.5048)
  line L2657 (23.7998, 75.9181) -> (24.4602, 75.9181)
  line L2658 (25.0469, 77.1652) -> (25.0469, 77.1652)
  line L2659 (24.9718, 77.3466) -> (24.6416, 77.6768)
  line L2660 (23.6184, 75.9932) -> (23.6184, 75.9932)
  line L2661 (23.7998, 75.9181) -> (23.7998, 75.9181)
  line L2662 (24.5584, 77.7324) -> (24.4602, 77.7519)
  line L2663 (23.2882, 76.3234) -> (23.6184, 75.9932)
  line L2664 (24.4602, 75.9181) -> (24.5584, 75.9376)
  line L2665 (24.4602, 75.9181) -> (24.4602, 75.9181)
  line L2666 (23.7016, 77.7324) -> (23.6184, 77.6768)
  line L2667 (24.4602, 77.7519) -> (24.4602, 77.7519)
  line L2668 (24.6416, 77.6768) -> (24.5584, 77.7324)
  line L2669 (25.0274, 76.4066) -> (25.0469, 76.5048)
  line L2670 (23.2882, 77.3466) -> (23.2882, 77.3466)
  line L2671 (23.2882, 76.3234) -> (23.2882, 76.3234)
  line L2672 (23.6184, 77.6768) -> (23.6184, 77.6768)
  line L2673 (23.6184, 77.6768) -> (23.2882, 77.3466)
  line L2674 (25.0469, 76.5048) -> (25.0469, 77.1652)
  line L2675 (23.2326, 76.4066) -> (23.2882, 76.3234)
  line L2676 (23.2326, 77.2634) -> (23.2131, 77.1652)
  line L2677 (23.6184, 75.9932) -> (23.7016, 75.9376)
  line L2678 (23.2131, 77.1652) -> (23.2131, 77.1652)
  line L2679 (25.0469, 76.5048) -> (25.0469, 76.5048)
  line L2680 (23.2882, 77.3466) -> (23.2326, 77.2634)
  line L2681 (27.0002, 75.9181) -> (27.0002, 75.9181)
  line L2682 (25.8282, 77.3466) -> (25.7726, 77.2634)
  line L2683 (25.7531, 76.5048) -> (25.7531, 76.5048)
  line L2684 (27.0002, 75.9181) -> (27.0984, 75.9376)
  line L2685 (26.1584, 77.6768) -> (25.8282, 77.3466)
  line L2686 (25.7531, 77.1652) -> (25.7531, 76.5048)
  line L2687 (26.2416, 77.7324) -> (26.1584, 77.6768)
  line L2688 (27.0002, 77.7519) -> (26.3398, 77.7519)
  line L2689 (27.5869, 76.5048) -> (27.5869, 76.5048)
  line L2690 (27.5869, 76.5048) -> (27.5869, 77.1652)
  line L2691 (27.5869, 77.1652) -> (27.5869, 77.1652)
  line L2692 (25.8282, 77.3466) -> (25.8282, 77.3466)
  line L2693 (26.1584, 77.6768) -> (26.1584, 77.6768)
  line L2694 (27.1816, 77.6768) -> (27.0984, 77.7324)
  line L2695 (27.1816, 75.9932) -> (27.1816, 75.9932)
  line L2696 (25.8282, 76.3234) -> (25.8282, 76.3234)
  line L2697 (27.5118, 77.3466) -> (27.1816, 77.6768)
  line L2698 (26.3398, 75.9181) -> (26.3398, 75.9181)
  line L2699 (26.2416, 75.9376) -> (26.3398, 75.9181)
  line L2700 (27.5118, 77.3466) -> (27.5118, 77.3466)
  line L2701 (26.3398, 75.9181) -> (27.0002, 75.9181)
  line L2702 (27.5118, 76.3234) -> (27.5118, 76.3234)
  line L2703 (26.1584, 75.9932) -> (26.2416, 75.9376)
  line L2704 (25.8282, 76.3234) -> (26.1584, 75.9932)
  line L2705 (25.7531, 77.1652) -> (25.7531, 77.1652)
  line L2706 (26.3398, 77.7519) -> (26.2416, 77.7324)
  line L2707 (27.5869, 77.1652) -> (27.5674, 77.2634)
  line L2708 (27.1816, 75.9932) -> (27.5118, 76.3234)
  line L2709 (27.0984, 77.7324) -> (27.0002, 77.7519)
  line L2710 (27.5674, 77.2634) -> (27.5118, 77.3466)
  line L2711 (26.1584, 75.9932) -> (26.1584, 75.9932)
  line L2712 (25.7726, 76.4066) -> (25.8282, 76.3234)
  line L2713 (25.7531, 76.5048) -> (25.7726, 76.4066)
  line L2714 (27.1816, 77.6768) -> (27.1816, 77.6768)
  line L2715 (25.7726, 77.2634) -> (25.7531, 77.1652)
  line L2716 (27.0002, 77.7519) -> (27.0002, 77.7519)
  line L2717 (27.0984, 75.9376) -> (27.1816, 75.9932)
  line L2718 (27.5118, 76.3234) -> (27.5674, 76.4066)
  line L2719 (26.3398, 77.7519) -> (26.3398, 77.7519)
  line L2720 (27.5674, 76.4066) -> (27.5869, 76.5048)
  line L2721 (76.5302, 75.2831) -> (76.6284, 75.3026)
  line L2722 (75.3582, 75.6884) -> (75.3582, 75.6884)
  line L2723 (75.2831, 75.8698) -> (75.2831, 75.8698)
  line L2724 (75.8698, 75.2831) -> (76.5302, 75.2831)
  line L2725 (75.3026, 75.7716) -> (75.3582, 75.6884)
  line L2726 (76.5302, 77.1169) -> (75.8698, 77.1169)
  line L2727 (75.6884, 75.3582) -> (75.6884, 75.3582)
  line L2728 (77.0418, 76.7116) -> (76.7116, 77.0418)
  line L2729 (77.1169, 75.8698) -> (77.1169, 75.8698)
  line L2730 (77.0418, 75.6884) -> (77.0418, 75.6884)
  line L2731 (76.6284, 77.0974) -> (76.5302, 77.1169)
  line L2732 (75.7716, 75.3026) -> (75.8698, 75.2831)
  line L2733 (75.2831, 76.5302) -> (75.2831, 76.5302)
  line L2734 (77.1169, 76.5302) -> (77.0974, 76.6284)
  line L2735 (76.5302, 77.1169) -> (76.5302, 77.1169)
  line L2736 (75.8698, 77.1169) -> (75.8698, 77.1169)
  line L2737 (75.6884, 77.0418) -> (75.3582, 76.7116)
  line L2738 (75.8698, 77.1169) -> (75.7716, 77.0974)
  line L2739 (75.3582, 76.7116) -> (75.3026, 76.6284)
  line L2740 (77.0974, 76.6284) -> (77.0418, 76.7116)
  line L2741 (77.1169, 75.8698) -> (77.1169, 76.5302)
  line L2742 (77.0418, 75.6884) -> (77.0974, 75.7716)
  line L2743 (76.7116, 77.0418) -> (76.7116, 77.0418)
  line L2744 (76.6284, 75.3026) -> (76.7116, 75.3582)
  line L2745 (77.0974, 75.7716) -> (77.1169, 75.8698)
  line L2746 (77.1169, 76.5302) -> (77.1169, 76.5302)
  line L2747 (75.3582, 76.7116) -> (75.3582, 76.7116)
  line L2748 (75.7716, 77.0974) -> (75.6884, 77.0418)
  line L2749 (75.6884, 77.0418) -> (75.6884, 77.0418)
  line L2750 (77.0418, 76.7116) -> (77.0418, 76.7116)
  line L2751 (75.2831, 75.8698) -> (75.3026, 75.7716)
  line L2752 (75.6884, 75.3582) -> (75.7716, 75.3026)
  line L2753 (76.5302, 75.2831) -> (76.5302, 75.2831)
  line L2754 (76.7116, 75.3582) -> (76.7116, 75.3582)
  line L2755 (75.2831, 76.5302) -> (75.2831, 75.8698)
  line L2756 (75.3026, 76.6284) -> (75.2831, 76.5302)
  line L2757 (75.3582, 75.6884) -> (75.6884, 75.3582)
  line L2758 (75.8698, 75.2831) -> (75.8698, 75.2831)
  line L2759 (76.7116, 77.0418) -> (76.6284, 77.0974)
  line L2760 (76.7116, 75.3582) -> (77.0418, 75.6884)
  line L2761 (4.635, 10.795) -> (2.3775, 10.795)
  line L2762 (4.635, 10.795) -> (6.8925, 10.795)
  line L2763 (4.635, 10.795) -> (4.635, 12.0025)
  line L2764 (4.635, 10.795) -> (4.635, 9.5875)
  line L2765 (12.7, 16.51) -> (11.8821, 16.51)
  line L2766 (12.7, 16.51) -> (13.5179, 16.51)
  line L2767 (12.7, 16.51) -> (12.7, 17.3279)
  line L2768 (12.7, 16.51) -> (12.7, 15.6921)
  line L2769 (15.875, 4.89) -> (15.875, 7.1475)
  line L2770 (15.875, 4.89) -> (15.875, 2.6325)
  line L2771 (15.875, 4.89) -> (17.0825, 4.89)
  line L2772 (15.875, 4.89) -> (14.6675, 4.89)
  line L2773 (24.13, 76.835) -> (23.3121, 76.835)
  line L2774 (24.13, 76.835) -> (24.9479, 76.835)
  line L2775 (24.13, 76.835) -> (24.13, 77.6529)
  line L2776 (24.13, 76.835) -> (24.13, 76.0171)
  line L2777 (25.4, 16.51) -> (24.5821, 16.51)
  line L2778 (25.4, 16.51) -> (26.2179, 16.51)
  line L2779 (25.4, 16.51) -> (25.4, 17.3279)
  line L2780 (25.4, 16.51) -> (25.4, 15.6921)
  line L2781 (26.67, 76.835) -> (27.4879, 76.835)
  line L2782 (26.67, 76.835) -> (25.8521, 76.835)
  line L2783 (26.67, 76.835) -> (26.67, 76.0171)
  line L2784 (26.67, 76.835) -> (26.67, 77.6529)
  line L2785 (28.575, 4.89) -> (28.575, 7.1475)
  line L2786 (28.575, 4.89) -> (28.575, 2.6325)
  line L2787 (28.575, 4.89) -> (29.7825, 4.89)
  line L2788 (28.575, 4.89) -> (27.3675, 4.89)
  line L2789 (38.1, 16.51) -> (37.2821, 16.51)
  line L2790 (38.1, 16.51) -> (38.9179, 16.51)
  line L2791 (38.1, 16.51) -> (38.1, 17.3279)
  line L2792 (38.1, 16.51) -> (38.1, 15.6921)
  line L2793 (41.275, 4.89) -> (41.275, 7.1475)
  line L2794 (41.275, 4.89) -> (41.275, 2.6325)
  line L2795 (41.275, 4.89) -> (42.4825, 4.89)
  line L2796 (41.275, 4.89) -> (40.0675, 4.89)
  line L2797 (48.895, 16.51) -> (48.0771, 16.51)
  line L2798 (48.895, 16.51) -> (49.7129, 16.51)
  line L2799 (48.895, 16.51) -> (48.895, 17.3279)
  line L2800 (48.895, 16.51) -> (48.895, 15.6921)
  line L2801 (53.34, 75.375) -> (53.34, 77.6325)
  line L2802 (53.34, 75.375) -> (53.34, 73.1175)
  line L2803 (53.34, 75.375) -> (54.5475, 75.375)
  line L2804 (53.34, 75.375) -> (52.1325, 75.375)
  line L2805 (54.61, 4.89) -> (54.61, 7.1475)
  line L2806 (54.61, 4.89) -> (54.61, 2.6325)
  line L2807 (54.61, 4.89) -> (55.8175, 4.89)
  line L2808 (54.61, 4.89) -> (53.4025, 4.89)
  line L2809 (54.61, 16.51) -> (55.4279, 16.51)
  line L2810 (54.61, 16.51) -> (53.7921, 16.51)
  line L2811 (54.61, 16.51) -> (54.61, 15.6921)
  line L2812 (54.61, 16.51) -> (54.61, 17.3279)
  line L2813 (64.77, 16.51) -> (65.5879, 16.51)
  line L2814 (64.77, 16.51) -> (63.9521, 16.51)
  line L2815 (64.77, 16.51) -> (64.77, 15.6921)
  line L2816 (64.77, 16.51) -> (64.77, 17.3279)
  line L2817 (67.31, 4.89) -> (67.31, 7.1475)
  line L2818 (67.31, 4.89) -> (67.31, 2.6325)
  line L2819 (67.31, 4.89) -> (68.5175, 4.89)
  line L2820 (67.31, 4.89) -> (66.1025, 4.89)
  line L2821 (76.2, 76.2) -> (77.0179, 76.2)
  line L2822 (76.2, 76.2) -> (75.3821, 76.2)
  line L2823 (76.2, 76.2) -> (76.2, 75.3821)
  line L2824 (76.2, 76.2) -> (76.2, 77.0179)
  line L2825 (76.2, 16.51) -> (77.0179, 16.51)
  line L2826 (76.2, 16.51) -> (75.3821, 16.51)
  line L2827 (76.2, 16.51) -> (76.2, 15.6921)
  line L2828 (76.2, 16.51) -> (76.2, 17.3279)
  line L2829 (80.01, 4.89) -> (80.01, 7.1475)
  line L2830 (80.01, 4.89) -> (80.01, 2.6325)
  line L2831 (80.01, 4.89) -> (81.2175, 4.89)
  line L2832 (80.01, 4.89) -> (78.8025, 4.89)
  line L2833 (87.63, 16.51) -> (88.4479, 16.51)
  line L2834 (87.63, 16.51) -> (86.8121, 16.51)
  line L2835 (87.63, 16.51) -> (87.63, 15.6921)
  line L2836 (87.63, 16.51) -> (87.63, 17.3279)
  line L2837 (95.44, 10.795) -> (93.1825, 10.795)
  line L2838 (95.44, 10.795) -> (97.6975, 10.795)
  line L2839 (95.44, 10.795) -> (95.44, 12.0025)
  line L2840 (95.44, 10.795) -> (95.44, 9.5875)
  line L2841 (54.61, 10.795) -> (54.61, 4.89)
  line L2842 (77.47, 10.795) -> (80.01, 10.795)
  line L2843 (80.01, 10.795) -> (88.265, 10.795)
  line L2844 (77.47, 10.795) -> (76.2, 10.795)
  line L2845 (76.2, 10.795) -> (67.31, 10.795)
  line L2846 (67.31, 10.795) -> (66.04, 10.795)